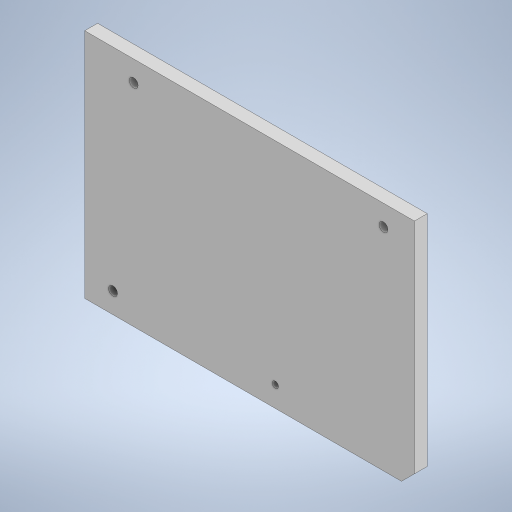
# Autodesk Inventor part: 아크릴 커버
Saved by Autodesk Inventor 2023 (Build 270158000, 158)
## iProperties
Created: 2022-11-10
Part Number: 아크릴 커버
Material: 일반
Document SubType Name: Modeling
Designer: user
Density: 1 g/cm^3
Appearance: 기본값
Author: user
Autodesk Inventor part; units mm, degrees
ref_plane "YZ Plane" through (0, 0, 0) normal (1, 0, 0) x (0, 1, 0)
ref_plane "XZ Plane" through (0, 0, 0) normal (0, 1, 0) x (-1, 0, 0)
ref_plane "XY Plane" through (0, 0, 0) normal (0, 0, 1) x (1, 0, 0)
sketch "스케치1" plane through (0, 0, 0) normal (0, 0, 1) x (1, 0, 0)
  line L0 (-64, 45) -> (64, 45)
  line L1 (64, 45) -> (64, -40)
  line L2 (59, -45) -> (-64, -45)
  line L3 (-64, -45) -> (-64, 45)
  line L4 (-64, 45) -> (64, -45) construction
  line L5 (64, 45) -> (-64, -45) construction
  line L6 (59, -45) -> (64, -40)
  circle A0 centre (-53, -37) radius 1.75
  circle A1 centre (10, -37) radius 1.25
  circle A2 centre (-45, 37) radius 1.75
  circle A3 centre (52, 37) radius 1.75
  point P0 (0, 0)
  dimension "d0" = 128
  dimension "d1" = 90
  dimension "d2" = 5
  dimension "d3" = 5
  dimension "d4" = 3.5
  dimension "d5" = 2.5
  dimension "d6" = 3.5
  dimension "d7" = 3.5
  dimension "d8" = 19
  dimension "d9" = 97
  dimension "d10" = 8
  dimension "d11" = 63
  dimension "d12" = 11
  dimension "d13" = 8
  constraints: 14 end point, 4 centre point, 2 horizontal alignment, 2 midpoint, 2 parallel, 2 point on line, 1 horizontal, 1 perpendicular
  measures "d0" distance of L0.start L0.end
  measures "d1" distance of L0.end L4.end
  measures "d2" distance of L2.start L4.end
  measures "d3" distance of L1.end L4.end
  measures "d4" diameter of A0
  measures "d5" diameter of A1
  measures "d6" diameter of A2
  measures "d7" diameter of A3
  measures "d8" distance from line of L3 A2.centre
  measures "d9" distance of A3.centre A2.centre
  measures "d10" distance from line of L0 A2.centre
  measures "d11" distance of A1.centre A0.centre
  measures "d12" distance from line of L3 A0.centre
  measures "d13" distance from line of L2 A0.centre
extrude "돌출1" add sketch "스케치1" along normal blind 5
equation "\"d3\" = d2"
